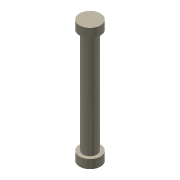
# Autodesk Inventor part: latchpin
Saved by Autodesk Inventor 2022 Beta2 (Build 260130000, 130) ContinuousBuild 0
## iProperties
Shininess: 64.0
Length Units: 11272
Angle Units: 11279
Time Units: 11290
Mass Units: 11286
Length Display Precision: 3
Angle Display Precision: 2
Created: 2002-01-23
Part Number: latchpin
Description: .7" long
Vendor: Pins R Us
Document SubType Name: Modeling
Designer: Administrator
Density: 1 g/cm^3
Material: Generic
Appearance: Light Beige
Density: 0.0
Volumn: 0.0
Area: 0.0
PropertySet Name: Model Information
Control State: 0
Master: False
Checked Out: False
Author: Administrator
Autodesk Inventor part; units mm, degrees
ref_plane "YZ Plane" through (0, 0, 0) normal (1, 0, 0) x (0, 1, 0)
ref_plane "XZ Plane" through (0, 0, 0) normal (0, 1, 0) x (-1, 0, 0)
ref_plane "XY Plane" through (0, 0, 0) normal (0, 0, 1) x (1, 0, 0)
sketch "Sketch1" plane through (0, 0, 0) normal (0, 0, 1) x (1, 0, 0)
  line L0 (-16.1234, 13.5158) -> (-16.1234, -4.2642)
  line L1 (-16.1234, -4.2642) -> (-14.5994, -4.2642)
  line L2 (-14.5994, -4.2642) -> (-14.5994, -2.9942)
  line L3 (-14.5994, -2.9942) -> (-15.1074, -2.9942)
  line L4 (-15.1074, -2.9942) -> (-15.1074, 12.2458)
  line L5 (-15.1074, 12.2458) -> (-14.5994, 12.2458)
  line L6 (-14.5994, 12.2458) -> (-14.5994, 13.5158)
  line L7 (-14.5994, 13.5158) -> (-16.1234, 13.5158)
  dimension "d0" = 1.27
  dimension "d1" = 17.78
  dimension "d2" = 1.524
  dimension "d3" = 0.508
  constraints: 16 end point, 6 parallel, 2 equal length, 1 perpendicular, 1 vertical
  measures "d0" distance of L1.end L2.end
  measures "d1" distance of L0.start L0.end
  measures "d2" distance of L0.end L1.end
  measures "d3" distance of L2.end L3.end
revolve "Revolution1" add sketch "Sketch1" angle 360 about axis through (-16.1234, 13.5158, 0) along (0, -1, 0)
body "Solid1"
